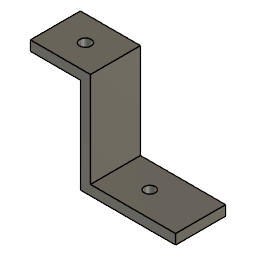
mocowanie_czujnik (Autodesk Fusion 360 design; units mm, degrees)
part number: 2025-11-28-17-20-17-522
part number: 2025-11-28-17-33-48-723
Autodesk Fusion 360 part; units mm, degrees
other "Kontekst pochodny1"
sketch "Szkic1" plane through (0, 0, 0) normal (0, 0, 1) x (1, 0, 0)
  line L0 (0, 0) -> (12, 0)
  line L1 (12, 0) -> (12, -19)
  line L2 (12, -19) -> (29, -19)
  line L3 (29, -19) -> (29, -21)
  line L4 (29, -21) -> (10, -21)
  line L5 (10, -21) -> (10, -2)
  line L6 (10, -2) -> (0, -2)
  line L7 (0, -2) -> (0, 0)
  dimension "d1" = 12
  dimension "d2" = 19
  dimension "d3" = 17
  dimension "d4" = 2
  dimension "d5" = 19
  dimension "d6" = 19
  dimension "d7" = 10
  dimension "d8" = 2
  constraint coincident L0.start L7.end
  constraint horizontal L0
  constraint perpendicular L0 L1
  constraint perpendicular L1 L2
  constraint perpendicular L2 L3
  constraint perpendicular L3 L4
  constraint vertical L5
  constraint perpendicular L5 L6
  measures "d1" distance of L0.start L0.end
  measures "d2" distance of L0.end L1.end
  measures "d3" distance of L1.end L2.end
  measures "d4" distance of L2.end L3.end
  measures "d5" distance of L3.end L4.end
  measures "d6" distance of L4.end L5.end L2.end
  measures "d7" distance of L5.end L6.end L2.end
  measures "d8" distance of L6.end L0.start
extrude "Wyciągnięcie proste1" add sketch "Szkic1" along normal blind 10 makes body 1
copy_body "Bryła->Komponent1" bodies 1 removing the originals makes body 2 in component "Component"
move_body "Przesuń1" bodies 2 to x (1, 0, 0) y (0, 0, 1) z (0, -1, 0) at (0, -21, 21) in component "Component"
sketch "Szkic2" plane through (0, 0, 0) normal (0, 0, 1) x (1, 0, 0)
  line L0 (29, -21) -> (29, -26) construction
  line L1 (29, -26) -> (18.84, -26) construction
  circle A0 centre (18.84, -26) radius 1.092
  dimension "d11" = 5
  dimension "d12" = 10.16
  dimension "d13" = 2.184
  constraint vertical L0
  constraint perpendicular L0 L1
  constraint coincident L1.end A0.centre
  measures "d11" distance of L0.start L0.end
  measures "d12" distance of L0.end L1.end
  measures "d13" diameter of A0
extrude "Wyciągnięcie proste1'" cut sketch "Szkic2" along normal blind 2 bodies 2 in component "Component"
sketch "Szkic3" plane through (0, 0, 21) normal (0, 0, 1) x (-1, 0, 0)
  line L0 (-12, 21) -> (0, 21)
  line L1 (0, 21) -> (0, 31)
  line L2 (0, 31) -> (-12, 31)
  line L3 (-12, 31) -> (-12, 21)
  line L4 (-12, 31) -> (0, 21) construction
  line L5 (-12, 21) -> (0, 31) construction
  circle A0 centre (-6, 26) radius 1.15
  dimension "d16" = 2.3
  constraint coincident L2.end L3.start
  constraint coincident L0.end L1.start
  constraint coincident L0.start L3.end
  constraint coincident L1.end L2.start
  constraint midpoint L5 A0.centre
  measures "d16" diameter of A0
extrude "Wyciągnięcie proste2" cut sketch "Szkic3" against normal blind 2 contours A0 bodies 2 in component "Component"
component "Component" placed x (1, 0, 0) y (0, 1, 0) z (0, 0, 1) at (0, 0, 0)
